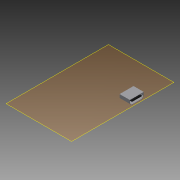
# Autodesk Inventor part: nanopc_t4_hdmi
Saved by Autodesk Inventor 2013 SP2 (Build 170200200, 200)
## iProperties
Created: 2018-09-03
Part Number: nanopc_t4_hdmi
Material: Generic
Document SubType Name: Modeling
Designer: alex
Density: 1 g/cm^3
Mass: 0.256489 g
Surface Area: 12.2368 cm^2
Volume: 0.256489 cm^3
Author: alex
Autodesk Inventor part; units mm, degrees
ref_plane "YZ Plane" through (0, 0, 0) normal (1, 0, 0) x (0, 1, 0)
ref_plane "XZ Plane" through (0, 0, 0) normal (0, 1, 0) x (-1, 0, 0)
ref_plane "XY Plane" through (0, 0, 0) normal (0, 0, 1) x (1, 0, 0)
ref_plane "Work Plane2" through (0, 0, 0) normal (0, 0, 1) x (1, 0, 0)
sketch "Sketch1" plane through (0, 0, 0) normal (0, 0, 1) x (1, 0, 0)
  line L0 (22.4943, 24.3103) -> (33.4943, 24.3103)
  line L1 (33.4943, 24.3103) -> (33.4943, 9.3103)
  line L2 (33.4943, 9.3103) -> (22.4943, 9.3103)
  line L3 (22.4943, 9.3103) -> (22.4943, 24.3103)
  point P0 (0, 0)
  dimension "d0" = 11
  dimension "d2" = 15
  constraints: 8 end point, 2 parallel, 1 horizontal, 1 perpendicular
  measures "d0" distance of L1.end L2.end
  measures "d2" distance of L0.end L1.end
extrude "Extrusion1" add sketch "Sketch1" along normal blind 5.6
chamfer "Chamfer1" distance 2 angle 45 2 edges at (27.9943, 9.3103, 0) (27.9943, 24.3103, 0)
shell "Shell1" thickness 0.3 removed faces 1 at (33.4943, 18.6436, 3.7333)
sketch "Sketch2" plane through (22.7943, 9.6103, 5.3) normal (1, 0, 0) x (0, 0, -1)
  line L0 (3.1757, 14.4) -> (0, 14.4) projected
  line L1 (0, 14.4) -> (0, 0) projected
  line L2 (3.1757, 0) -> (0, 0) projected
  line L3 (2.6, 12.4) -> (1.6, 12.4)
  line L4 (1.6, 12.4) -> (1.6, 2)
  line L5 (1.6, 2) -> (2.6, 2)
  line L6 (2.6, 2) -> (2.6, 12.4)
  point P0 (5.3, -9.6103)
  dimension "d9" = 1
  dimension "d12" = 2
  dimension "d13" = 2
  dimension "d14" = 1.6
  constraints: 8 end point, 2 parallel, 1 horizontal, 1 perpendicular
  measures "d9" distance of L3.start L3.end
  measures "d12" distance between parallel lines of L0 L3
  measures "d13" distance between parallel lines of L2 L5
  measures "d14" distance between parallel lines of L1 L4
extrude "Extrusion2" add sketch "Sketch2" along normal up to surface (10.7 mm away)
body "Solid1"
